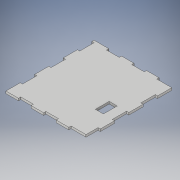
# Autodesk Inventor part: KANAN
Saved by Autodesk Inventor 2019 (Build 230136000, 136)
## iProperties
Created: 2019-11-24
Part Number: KANAN
Material: Generic
Document SubType Name: Modeling
Designer: User
Density: 1 g/cm^3
Appearance: Default
Author: User
Autodesk Inventor part; units mm, degrees
ref_plane "YZ Plane" through (0, 0, 0) normal (1, 0, 0) x (0, 1, 0)
ref_plane "XZ Plane" through (0, 0, 0) normal (0, 1, 0) x (-1, 0, 0)
ref_plane "XY Plane" through (0, 0, 0) normal (0, 0, 1) x (1, 0, 0)
sketch "Sketch1" plane through (0, 0, 0) normal (0, 1, 0) x (-1, 0, 0)
  line L0 (34, 37.5) -> (-34, -37.5) construction
  line L1 (-34, 37.5) -> (34, -37.5) construction
  line L2 (34, 37.5) -> (34, 25)
  line L3 (34, 25) -> (32, 25)
  line L4 (32, 25) -> (32, 12.5)
  line L5 (32, 12.5) -> (34, 12.5)
  line L6 (34, 12.5) -> (34, 0)
  line L7 (34, 0) -> (32, 0)
  line L8 (32, 0) -> (32, -12.5)
  line L9 (32, -12.5) -> (34, -12.5)
  line L10 (34, -12.5) -> (34, -25)
  line L11 (34, -25) -> (32, -25)
  line L12 (32, -25) -> (32, -37.5)
  line L13 (34, -25) -> (34, -12.5)
  line L14 (34, 0) -> (34, 12.5)
  line L15 (34, 25) -> (34, 37.5)
  line L16 (32, -39.5) -> (21, -39.5)
  line L17 (21, -39.5) -> (21, -37.5)
  line L18 (21, -37.5) -> (10, -37.5)
  line L19 (10, -37.5) -> (10, -39.5)
  line L20 (10, -39.5) -> (-1, -39.5)
  line L21 (-1, -39.5) -> (-1, -37.5)
  line L22 (-1, -37.5) -> (-12, -37.5)
  line L23 (-12, -37.5) -> (-12, -39.5)
  line L24 (-12, -39.5) -> (-23, -39.5)
  line L25 (-36, -37.5) -> (-36, -25)
  line L26 (-36, -25) -> (-34, -25)
  line L27 (-34, -25) -> (-34, -12.5)
  line L28 (-34, -12.5) -> (-36, -12.5)
  line L29 (-36, -12.5) -> (-36, 0)
  line L30 (-36, 0) -> (-34, 0)
  line L31 (-34, 0) -> (-34, 12.5)
  line L32 (-34, 12.5) -> (-34, 8.9552)
  line L33 (-34, 12.5) -> (-36, 12.5)
  line L34 (-36, 12.5) -> (-36, 25)
  line L35 (-36, 25) -> (-34, 25)
  line L36 (10, -37.5) -> (21, -37.5)
  line L37 (-34, -37.5) -> (-24.5, -37.5)
  line L38 (-12, -37.5) -> (-1, -37.5)
  line L39 (-34, -12.5) -> (-34, -25)
  line L40 (-34, 35.5) -> (-34, 25)
  line L41 (-34, 12.5) -> (-34, 0)
  line L42 (34, 37.5) -> (23, 37.5)
  line L43 (23, 37.5) -> (23, 35.5)
  line L44 (23, 35.5) -> (12, 35.5)
  line L45 (12, 35.5) -> (12, 37.5)
  line L46 (12, 37.5) -> (1, 37.5)
  line L47 (1, 37.5) -> (1, 35.5)
  line L48 (1, 35.5) -> (-10, 35.5)
  line L49 (-10, 35.5) -> (-10, 37.5)
  line L50 (-10, 37.5) -> (-21, 37.5)
  line L51 (-21, 37.5) -> (-21, 35.5)
  line L52 (-21, 35.5) -> (-34, 35.5)
  line L53 (34, 37.5) -> (23, 37.5)
  line L54 (12, 37.5) -> (1, 37.5)
  line L55 (-10, 37.5) -> (-21, 37.5)
  line L56 (-26, 12.25) -> (-19, 12.25)
  line L57 (-19, 12.25) -> (-19, 0.25)
  line L58 (-19, 0.25) -> (-26, 0.25)
  line L59 (-26, 0.25) -> (-26, 12.25)
  line L60 (-26, 12.25) -> (-19, 0.25) construction
  line L61 (-19, 12.25) -> (-26, 0.25) construction
  line L62 (32, -37.5) -> (34, -37.5)
  line L63 (34, -39.5) -> (32, -39.5)
  line L64 (34, -37.5) -> (34, -39.5)
  line L65 (-34, -37.5) -> (-36, -37.5)
  line L66 (-23, -39.5) -> (-23, -37.5)
  line L67 (-23, -37.5) -> (-24.5, -37.5)
  point P0 (0, 0)
  point P1 (-35.8133, -39.5)
  dimension "d3" = 2
  dimension "d4" = 12.5
  dimension "d5" = 12.5
  dimension "d6" = 12.5
  dimension "d7" = 12.5
  dimension "d11" = 11
  dimension "d12" = 11
  dimension "d13" = 11
  dimension "d14" = 11
  dimension "d17" = 12.5
  dimension "d18" = 2
  dimension "d19" = 12.5
  dimension "d20" = 12.5
  dimension "d21" = 2
  dimension "d22" = 12.5
  dimension "d23" = 11
  dimension "d26" = 11
  dimension "d28" = 11
  dimension "d29" = 11
  dimension "d32" = 7
  dimension "d33" = 12
  dimension "d36" = 13
  constraints: 136 end point, 44 perpendicular, 21 parallel, 14 point on line, 6 horizontal, 2 midpoint, 1 collinear, 1 vertical
  measures "d3" distance of L2.end L3.end
  measures "d4" distance of L3.end L4.end
  measures "d5" distance of L5.end L6.end
  measures "d6" distance of L7.end L8.end
  measures "d7" distance of L10.end L9.end
  measures "d11" distance of L17.end L18.end
  measures "d12" distance of L19.end L20.end
  measures "d13" distance of L21.end L22.end
  measures "d14" distance of L23.end L24.end
  measures "d17" distance of L26.end L27.end
  measures "d18" distance of L27.end L28.end
  measures "d19" distance of L28.end L29.end
  measures "d20" distance of L30.end L31.end
  measures "d21" distance of L31.end L33.end
  measures "d22" distance of L33.end L34.end
  measures "d23" distance of L0.start L42.end
  measures "d26" distance of L45.end L46.end
  measures "d28" distance of L47.end L48.end
  measures "d29" distance of L50.end L49.end
  measures "d32" distance of L57.end L58.end
  measures "d33" distance of L56.end L57.end
  measures "d36" distance between parallel lines of L25 L66
extrude "Extrusion1" add sketch "Sketch1" along normal blind 2
body "Solid1"
